AgriRover_Base (Autodesk Fusion 360 design; units mm, degrees)
part number: 2026-09-19-14-31-14-166
Autodesk Fusion 360 part; units mm, degrees
sketch "Sketch1" plane through (0, 0, 0) normal (0, 0, 1) x (1, 0, 0)
  line L0 (-50, 50) -> (200, 50)
  line L1 (200, 50) -> (200, -150)
  line L2 (200, -150) -> (-50, -150)
  line L3 (-50, -150) -> (-50, 50)
  line L4 (-55, 25) -> (-55, 51)
  line L5 (-55, 55) -> (-25, 55)
  line L6 (-51, 55) -> (201, 55)
  line L7 (205, 51) -> (205, -151)
  line L8 (201, -155) -> (-51, -155)
  line L9 (-55, -151) -> (-55, 55)
  arc A0 (-51, 55) -> (-55, 51) centre (-51, 51) ccw
  arc A1 (205, 51) -> (201, 55) centre (201, 51) ccw
  arc A2 (201, -155) -> (205, -151) centre (201, -151) ccw
  arc A3 (-55, -151) -> (-51, -155) centre (-51, -151) ccw
  point P0 (205, 55)
  point P1 (-55, -155)
  dimension "d1" = 250
  dimension "d2" = 200
  dimension "d3" = 260
  dimension "d4" = 210
  dimension "d5" = 4
  dimension "d6" = 4
  dimension "d7" = 4
  dimension "d8" = 4
  constraint horizontal L0
  constraint vertical L1
  constraint horizontal L2
  constraint vertical L3
  constraint parallel L3 L4
  constraint perpendicular L4 L5
  constraint horizontal L6
  constraint vertical L7
  constraint horizontal L8
  constraint vertical L9
  constraint coincident L5.start L6
  constraint coincident L5.start L4
  constraint tangent L6 A0
  constraint tangent L4 A0
  constraint coincident P0 L6
  constraint coincident P0 L7
  constraint tangent L6 A1
  constraint tangent L7 A1
  constraint tangent L7 A2
  constraint tangent L8 A2
  constraint coincident P1 L9
  constraint coincident P1 L8
  constraint tangent L9 A3
  constraint tangent L8 A3
  measures "d1" distance of L0.start L0.end
  measures "d2" distance of L0.start L2.end
  measures "d3" distance of L5.start P0
  measures "d4" distance of L5.start P1
  measures "d5" radius of A0
  measures "d6" radius of A1
  measures "d7" radius of A2
  measures "d8" radius of A3
extrude "Extrude1" add sketch "Sketch1" along normal blind 50 contours L4 L5 L6 L7 L8 L9 A0 A1 A2 A3
sketch "Sketch2" plane through (0, 0, 0) normal (0, 0, -1) x (1, 0, 0)
  line L0 (-50, 150) -> (200, 150)
  line L1 (200, 150) -> (200, -50)
  line L2 (200, -50) -> (-50, -50)
  line L3 (-50, -50) -> (-50, 150)
  line L4 (-55, 151) -> (-55, -51)
  arc A0 (-55, -51) -> (-51, -55) centre (-51, -51) ccw
  line L5 (-51, -55) -> (201, -55)
  arc A1 (201, -55) -> (205, -51) centre (201, -51) ccw
  line L6 (205, -51) -> (205, 151)
  arc A2 (205, 151) -> (201, 155) centre (201, 151) ccw
  line L7 (201, 155) -> (-51, 155)
  arc A3 (-51, 155) -> (-55, 151) centre (-51, 151) ccw
sketch "Sketch3" plane through (0, 0, 0) normal (0, 0, -1) x (1, 0, 0)
  line L0 (-51, 155) -> (201, 155)
  line L1 (205, 151) -> (205, -51)
  line L2 (201, -55) -> (-51, -55)
  line L3 (-55, -51) -> (-55, 151)
  arc A0 (201, -55) -> (205, -51) centre (201, -51) ccw
  arc A1 (205, 151) -> (201, 155) centre (201, 151) ccw
  arc A2 (-51, 155) -> (-55, 151) centre (-51, 151) ccw
  arc A3 (-55, -51) -> (-51, -55) centre (-51, -51) ccw
  dimension "d11" = 4
  dimension "d12" = 4
  dimension "d13" = 4
  dimension "d14" = 4
  constraint horizontal L0
  constraint vertical L1
  constraint horizontal L2
  constraint vertical L3
  constraint tangent L2 A0
  constraint tangent L1 A0
  constraint tangent L1 A1
  constraint tangent L0 A1
  constraint tangent L0 A2
  constraint tangent L3 A2
  constraint tangent L3 A3
  constraint tangent L2 A3
  measures "d11" radius of A0
  measures "d12" radius of A1
  measures "d13" radius of A2
  measures "d14" radius of A3
extrude "Extrude2" add sketch "Sketch3" along normal blind 5
sketch "Sketch4" plane through (0, 0, 50) normal (0, 0, 1) x (-1, 0, 0)
  line L0 (-200, 150) -> (50, 150)
  line L1 (50, 150) -> (50, -50)
  line L2 (50, -50) -> (-200, -50)
  line L3 (-200, -50) -> (-200, 150)
  line L4 (55, -51) -> (55, 151)
  arc A0 (55, 151) -> (51, 155) centre (51, 151) ccw
  line L5 (51, 155) -> (-201, 155)
  arc A1 (-201, 155) -> (-205, 151) centre (-201, 151) ccw
  line L6 (-205, 151) -> (-205, -51)
  arc A2 (-205, -51) -> (-201, -55) centre (-201, -51) ccw
  line L7 (-201, -55) -> (51, -55)
  arc A3 (51, -55) -> (55, -51) centre (51, -51) ccw
  circle A4 centre (52, -52) radius 2
  circle A5 centre (-202, -52) radius 2
  circle A6 centre (-202, 152) radius 2
  circle A7 centre (52, 152) radius 2
  dimension "d17" = 4
  dimension "d18" = 4
  dimension "d19" = 4
  measures "d17" diameter of A5
  measures "d18" diameter of A6
  measures "d19" diameter of A7
extrude "Extrude3" cut sketch "Sketch4" against normal blind 10 contours A4 | A5 | A6 | A7
thread "Thread1" "ISO Metric profile 4.0 M4x0.7 M4x0.7 6H" major diameter 4.1095 minor diameter 3.332 pitch 0.7 angle 60 resizes the face on face at (200.0618, -152.4935, 43.3333)
thread "Thread2" "ISO Metric profile 4.0 M4x0.7 M4x0.7 6H" major diameter 4.1095 minor diameter 3.332 pitch 0.7 angle 60 resizes the face on face at (-52.5417, 50.0748, 43.3333) on face at (200.9149, 50.3199, 43.3333) on face at (-50.0618, -152.4935, 43.3333)
